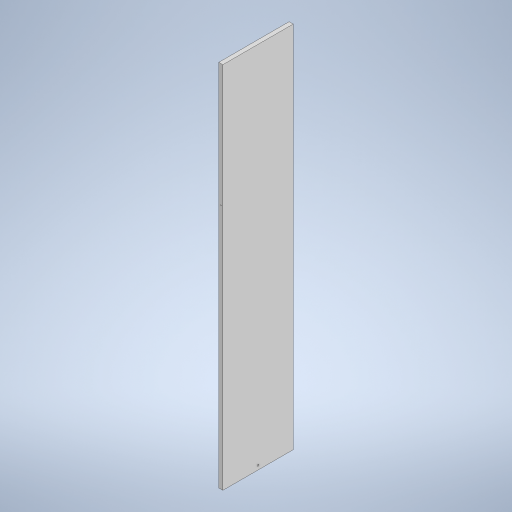
# Autodesk Inventor part: support_seed_holder
Saved by Autodesk Inventor 2023 (Build 270158000, 158)
## iProperties
Created: 2022-06-19
Part Number: support_seed_holder
Material: Generic
Document SubType Name: Modeling
Designer: prana_p9lsmih
Density: 1 g/cm^3
Appearance: Default
Author: prana_p9lsmih
Autodesk Inventor part; units mm, degrees
ref_plane "YZ Plane" through (0, 0, 0) normal (1, 0, 0) x (0, 1, 0)
ref_plane "XZ Plane" through (0, 0, 0) normal (0, 1, 0) x (-1, 0, 0)
ref_plane "XY Plane" through (0, 0, 0) normal (0, 0, 1) x (1, 0, 0)
sketch "Sketch1" plane through (0, 0, 0) normal (1, 0, 0) x (0, 1, 0)
  line L0 (0, 0) -> (450, 0)
  line L1 (450, 0) -> (450, -86)
  line L2 (450, -86) -> (0, -86)
  line L3 (0, -86) -> (0, 0)
  dimension "d0" = 450
  dimension "d1" = 86
  constraints: 8 end point, 2 parallel, 1 horizontal, 1 perpendicular
  measures "d0" distance of L1.end L2.end
  measures "d1" distance of L0.end L1.end
extrude "Extrusion1" add sketch "Sketch1" along normal blind 5
sketch "Sketch2" plane through (5, 0, 0) normal (1, 0, 0) x (0, 0, -1)
  line L0 (0, 0) -> (86, 0) projected
  line L1 (0, 450) -> (0, 0) projected
  point P0 (43, 5)
  dimension "d4" = 5
  dimension "d5" = 43
  measures "d4" distance from line of L0 point (43, 5)
  measures "d5" distance from line of L1 point (43, 5)
hole "Hole1" at (5, 5, -43) direction (-1, 0, 0) diameter 2 end through all
sketch "Sketch3" plane through (0, 0, 0) normal (0, 0, 1) x (1, 0, 0)
  line L0 (0, 450) -> (5, 450) projected
  line L1 (5, 450) -> (5, 0) projected
  point P0 (0, 0)
  point P1 (2.5, 300)
  dimension "d13" = 150
  dimension "d14" = 2.5
  measures "d13" distance from line of L0 point (2.5, 300)
  measures "d14" distance from line of L1 point (2.5, 300)
hole "Hole2" at (2.5, 300, 0) direction (0, 0, -1) diameter 1 end through all
body "Solid1"
